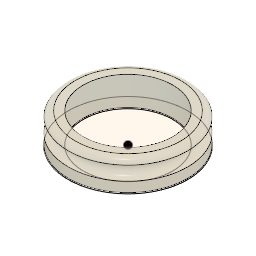
male_socket (Autodesk Fusion 360 design; units mm, degrees)
Autodesk Fusion 360 part; units mm, degrees
note: some values were not read from the file. Set by a fixed rule: which sketch regions a step uses.
sketch "Sketch1" plane through (0, 0, 0) normal (0, 1, 0) x (1, 0, 0)
  circle A0 centre (0, 0) radius 12
  circle A1 centre (0, 0) radius 9
  dimension "d1" = 24
  dimension "d2" = -3
  constraint coincident A0.centre A1.centre
  measures "d1" diameter of A0
sketch "Sketch2" plane through (0, 0, 0) normal (0, 0, 1) x (1, 0, 0)
  line L0 (9, 0) -> (12, 0)
  line L1 (12, 0) -> (12, 6)
  line L2 (12, 6) -> (9, 6)
  line L3 (9, 6) -> (9, 0)
  line L4 (9, 2.2) -> (12, 2.2) construction
  line L5 (9, 5) -> (12, 5) construction
  arc A0 (12, 5) -> (12, 2.2) centre (11.9033, 3.6) ccw
  line L6 (10.5, 3.6) -> (12, 3.6) construction
  line L7 (10.5, 6) -> (10.5, 0) construction
  dimension "d6" = 3
  dimension "d14" = 6
  dimension "d17" = 1
  dimension "d40" = 1.5
  dimension "d41" = 2.2
  constraint horizontal L0
  constraint vertical L1
  constraint horizontal L2
  constraint vertical L3
  constraint coincident L3 L4.start
  constraint coincident L1 L4.end
  constraint perpendicular L1 L4
  constraint coincident L3 L5.start
  constraint coincident L1 L5.end
  constraint perpendicular L1 L5
  constraint midpoint A0 L6.start
  constraint coincident L1 L6.end
  constraint perpendicular L1 L6
  constraint midpoint L2 L7.start
  constraint midpoint L0 L7.end
  measures "d6" distance of L1 L3
  measures "d14" distance of L0 L2
  measures "d17" distance of L2 L5
  measures "d40" distance of L3 L6.start
  measures "d41" distance of L0 L4
sweep "Sweep1" add profiles "Sketch2" path "Sketch1" along A1 section 1 contours L0 L1 L2 L3 A0
fillet "Fillet1" radius 1.5 1 edges at (-11.1879, 6, 4.3394)
extrude "Extrude1" cut sketch "Sketch1" along normal blind 0.2
